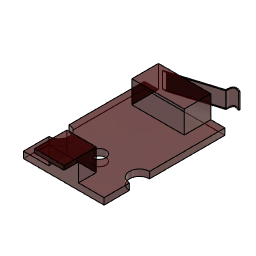
Rover base v7 (Autodesk Fusion 360 archive; units mm, degrees)
design "Crash sensor"
Autodesk Fusion 360 part; units mm, degrees
sketch "Sketch1" plane through (0, 0, 0) normal (0, 0, 1) x (1, 0, 0)
  line L0 (10, -15) -> (-10, -15)
  line L1 (-10, -15) -> (-10, 15)
  line L2 (-10, 15) -> (10, 15)
  line L3 (10, 15) -> (10, -15)
  line L4 (10, -15) -> (-10, 15) construction
  line L5 (-10, -15) -> (10, 15) construction
  dimension "d1" = 20
  dimension "d2" = 30
  constraint horizontal L0
  constraint perpendicular L0 L1
  constraint parallel L0 L2
  constraint parallel L1 L3
  constraint coincident L4 origin
  constraint coincident L5 origin
  measures "d1" distance of L1.end L2.end
  measures "d2" distance of L0.start L2.end
extrude "Extrude1" add sketch "Sketch1" along normal blind 1.6
sketch "Sketch2" plane through (0, 0, 1.6) normal (0, 0, 1) x (-1, 0, 0)
  line L0 (-10, -15) -> (10, -15)
  line L1 (10, -15) -> (10, 15)
  line L2 (10, 15) -> (-10, 15)
  line L3 (-10, 15) -> (-10, -15)
  line L4 (6.5, -15) -> (-6.5, -15)
  line L5 (-6.5, -15) -> (-6.5, -8.4)
  line L6 (-6.5, -8.4) -> (6.5, -8.4)
  line L7 (6.5, -8.4) -> (6.5, -15)
  point P0 (0, -8.4)
  dimension "d5" = 13
  dimension "d6" = 6.6
  constraint horizontal L4
  constraint vertical L5
  constraint horizontal L6
  constraint vertical L7
  constraint midpoint L6 P0
  constraint vertical origin P0
  constraint collinear L0 L4
  measures "d5" distance of L4.start L4.end
  measures "d6" distance of L4.end L5.end
extrude "Extrude2" add sketch "Sketch2" along normal blind 5.6 contours L0 L4 L5 L6 L7
sketch "Sketch3" plane through (0, 0, 7.2) normal (0, 0, 1) x (-1, 0, 0)
  line L0 (6.5, -8.4) -> (-6.5, -8.4)
  line L1 (-6.5, -8.4) -> (-6.5, -15)
  line L2 (-6.5, -15) -> (6.5, -15)
  line L3 (6.5, -15) -> (6.5, -8.4)
  line L4 (5.5056, -15) -> (-6.5, -18.7)
  spline S0 degree 5 poles (-6.5, -18.7) (-6.4971, -18.7969) (-6.4951, -18.9849) (-6.504, -19.2489) (-6.5399, -19.5646) (-6.6275, -19.8945) (-6.7616, -20.154) (-6.9462, -20.3373) (-7.1832, -20.441) (-7.4708, -20.4684) (-7.8051, -20.4252) (-8.1068, -20.3387) (-8.3512, -20.2464) (-8.522, -20.173) (-8.6094, -20.1333) knots 0 0 0 0 0 0 0.1 0.2 0.3 0.4 0.5 0.6 0.7 0.8 0.9 1 1 1 1 1 1
  line L5 (5.4173, -14.7133) -> (-6.8068, -18.4806)
  spline S1 degree 3 poles (-6.8068, -18.4806) (-6.8045, -18.5568) (-6.8022, -18.6329) (-6.7999, -18.7091) (-6.7803, -19.3532) (-6.8883, -19.803) (-7.0372, -19.9851) (-7.1506, -20.1238) (-7.2845, -20.1741) (-7.572, -20.1446) (-7.8085, -20.1203) (-8.1221, -20.0252) (-8.4853, -19.8601) knots -0.047137 -0.047137 -0.047137 -0.047137 0 0 0 0.418701 0.418701 0.418701 0.737623 0.737623 0.737623 1 1 1 1
  line L6 (-8.4853, -19.8601) -> (-8.6094, -20.1333)
  line L7 (5.4173, -14.7133) -> (5.5056, -15)
  point P0 (-6.9617, -20.3191)
  dimension "d9" = 3.7
  dimension "d10" = 0.3
  constraint coincident L2 L4.start
  constraint perpendicular L4 L7
  measures "d9" distance of L1.end L4.end
extrude "Extrude3" add sketch "Sketch3" against normal blind 4 from surface at -1 contours L2 L4 S0 L5 S1 L6
sketch "Sketch4" plane through (0, 0, 1.6) normal (0, 0, 1) x (-1, 0, 0)
  line L0 (-6.5, -15) -> (-6.5, -8.4)
  line L1 (-6.5, -8.4) -> (6.5, -8.4)
  line L2 (6.5, -8.4) -> (6.5, -15)
  line L3 (6.5, -15) -> (10, -15)
  line L4 (10, -15) -> (10, 15)
  line L5 (10, 15) -> (-10, 15)
  line L6 (-10, 15) -> (-10, -15)
  line L7 (-10, -15) -> (-6.5, -15)
  circle A0 centre (-10, 6.2) radius 2.5
  circle A1 centre (10, 6.2) radius 2.5
  circle A2 centre (0, 6.2) radius 1.65
  dimension "d14" = 5
  dimension "d15" = 5
  dimension "d16" = 8.8
  dimension "d17" = 8.8
  dimension "d18" = 3.3
  dimension "d19" = 8.8
  constraint coincident L6 A0.centre
  constraint coincident L4 A1.centre
  constraint vertical origin A2.centre
  measures "d14" diameter of A0
  measures "d15" diameter of A1
  measures "d16" distance of L5.end A0.centre
  measures "d17" distance of L4.end A1.centre
  measures "d18" diameter of A2
  measures "d19" distance of L5 A2.centre
extrude "Extrude4" cut sketch "Sketch4" against normal blind 6 contours L6 A0 | L4 A1 | A2 picked at (-9.2516, 6.7372) picked at (8.4513, 6.9963)
sketch "Sketch5" plane through (0, 0, 1.6) normal (0, 0, 1) x (-1, 0, 0)
  arc A0 (-10, 3.7) -> (-10, 8.7) centre (-10, 6.2) ccw
  line L0 (-10, 3.7) -> (-10, -15)
  line L1 (-10, -15) -> (-6.5, -15)
  line L2 (-6.5, -15) -> (-6.5, -8.4)
  line L3 (-6.5, -8.4) -> (6.5, -8.4)
  line L4 (6.5, -8.4) -> (6.5, -15)
  line L5 (6.5, -15) -> (10, -15)
  line L6 (10, -15) -> (10, 3.7)
  arc A1 (10, 8.7) -> (10, 3.7) centre (10, 6.2) ccw
  line L7 (10, 8.7) -> (10, 15)
  line L8 (10, 15) -> (-10, 15)
  line L9 (-10, 15) -> (-10, 8.7)
  circle A2 centre (0, 6.2) radius 1.65
  line L10 (3.65, 15) -> (-3.65, 15)
  line L11 (-3.65, 15) -> (-3.65, 10.58)
  line L12 (-3.65, 10.58) -> (3.65, 10.58)
  line L13 (3.65, 10.58) -> (3.65, 15)
  point P0 (0, 10.58)
  dimension "d22" = 4.42
  dimension "d23" = 7.3
  constraint horizontal L10
  constraint vertical L11
  constraint horizontal L12
  constraint vertical L13
  constraint coincident L8 L10.start
  constraint midpoint L12 P0
  constraint vertical origin P0
  measures "d2" distance of L0.end
  measures "d22" distance of L10.end L11.end
  measures "d23" distance of L10.start L10.end
extrude "Extrude5" add sketch "Sketch5" along normal blind 5.5 contours L8 L10 L11 L12 L13
sketch "Sketch6" plane through (0, 0, 7.1) normal (0, 0, 1) x (-1, 0, 0)
  line L0 (3.65, 10.58) -> (3.65, 15)
  line L1 (3.65, 15) -> (-3.65, 15)
  line L2 (-3.65, 15) -> (-3.65, 10.58)
  line L3 (-3.65, 10.58) -> (3.65, 10.58)
  line L4 (3.65, 10.58) -> (-3.65, 10.58)
  line L5 (-3.65, 10.58) -> (-3.65, 18.58)
  line L6 (-3.65, 18.58) -> (3.65, 18.58)
  line L7 (3.65, 18.58) -> (3.65, 10.58)
  dimension "d26" = 8
  constraint horizontal L4
  constraint vertical L5
  constraint horizontal L6
  constraint vertical L7
  constraint coincident L0.start L3.end
  constraint collinear L2 L5
  measures "d26" distance of L4 L6
extrude "Extrude6" add sketch "Sketch6" against normal blind 1 contours L1 L5 L6 L7

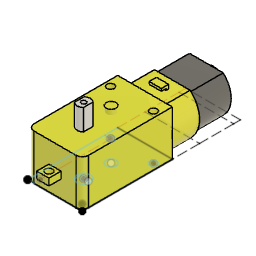
design "Yellow Gearbox motor v3"
Autodesk Fusion 360 part; units mm, degrees
sketch "Sketch1" plane through (0, 0, 0) normal (0, 0, 1) x (1, 0, 0) in component "Yellow TT Motor"
  line L0 (2.555, 0) -> (19.885, 0)
  line L1 (22.44, 2.555) -> (22.44, 37)
  line L2 (22.44, 37) -> (0, 37)
  line L3 (0, 37) -> (0, 2.555)
  arc A0 (19.885, 0) -> (22.44, 2.555) centre (19.885, 2.555) ccw
  arc A1 (0, 2.555) -> (2.555, 0) centre (2.555, 2.555) ccw
  line L4 (2.555, 2.555) -> (2.555, 11.805) construction
  circle A2 centre (11.22, 11.805) radius 0.975
  circle A3 centre (11.22, 11.805) radius 2.7
  line L5 (11.22, 11.805) -> (13.07, 11.805) construction
  line L6 (13.0698, 9.8382) -> (13.0698, 13.7718)
  line L7 (9.3702, 9.8382) -> (9.3702, 13.7718)
  line L8 (2.555, 11.805) -> (2.555, 23.055) construction
  line L9 (2.555, 23.055) -> (2.555, 31.655) construction
  line L10 (0, 31.655) -> (2.42, 31.655) construction
  line L11 (22.44, 31.655) -> (20.02, 31.655) construction
  circle A4 centre (2.42, 31.655) radius 1.5
  circle A5 centre (20.02, 31.655) radius 1.5
  circle A6 centre (11.22, 23.055) radius 2
  line L12 (0, 37) -> (0, 48.2) construction
  line L13 (0, 48.2) -> (22.44, 48.2) construction
  line L14 (22.44, 48.2) -> (22.44, 37) construction
  line L15 (0, 48.2) -> (0, 62.2) construction
  line L16 (0, 62.2) -> (22.44, 62.2) construction
  line L17 (22.44, 62.2) -> (22.44, 48.2) construction
  line L18 (22.44, 62.2) -> (22.44, 65) construction
  line L19 (22.44, 65) -> (0, 65) construction
  line L20 (0, 65) -> (0, 62.2) construction
  point P0 (22.44, 0)
  dimension "d1" = 22.44
  dimension "d2" = 37
  dimension "d3" = 2.555
  dimension "d5" = 9.25
  dimension "d6" = 1.95
  dimension "d7" = 5.4
  dimension "d8" = 1.85
  dimension "d10" = 11.25
  dimension "d11" = 8.6
  dimension "d13" = 2.42
  dimension "d14" = 3
  dimension "d15" = 3
  dimension "d16" = 4
  dimension "d28" = 11.2
  dimension "d29" = 14
  dimension "d45" = 2.8
  constraint horizontal L0
  constraint perpendicular L0 L1
  constraint perpendicular L1 L2
  constraint perpendicular L0 L3
  constraint coincident P0 L1
  constraint coincident P0 L0
  constraint tangent L1 A0
  constraint tangent L0 A0
  constraint coincident origin L0
  constraint tangent L3 A1
  constraint tangent L0 A1
  constraint equal A0 A1
  constraint coincident A1.centre L4.start
  constraint parallel L3 L4
  constraint concentric A2 A3
  constraint coincident A2.centre A3.centre
  constraint coincident A3 L6.start
  constraint coincident A3 L6.end
  constraint coincident A3 L7.start
  constraint coincident A3 L7.end
  constraint parallel L6 L7
  constraint parallel L3 L8
  constraint parallel L8 L9
  constraint coincident L3 L10.start
  constraint coincident L1 L11.start
  constraint perpendicular L9 L10
  constraint perpendicular L1 L11
  constraint coincident L10.end A4.centre
  constraint coincident L11.end A5.centre
  constraint perpendicular L2 L12
  constraint perpendicular L1 L13
  constraint perpendicular L2 L14
  constraint perpendicular L13 L15
  constraint perpendicular L14 L16
  constraint perpendicular L13 L17
  constraint perpendicular L16 L18
  constraint perpendicular L18 L19
  constraint perpendicular L16 L20
  measures "d1" distance of origin P0
  measures "d2" distance of P0 L1.end
  measures "d3" radius of A0
  measures "d5" distance of A1.centre L4.end
  measures "d6" diameter of A2
  measures "d7" diameter of A3
  measures "d8" distance of A2.centre L5.end
  measures "d10" distance of L4.end L8.end
  measures "d11" distance of L8.end L9.end
  measures "d13" distance of L11.start L11.end
  measures "d14" diameter of A4
  measures "d15" diameter of A5
  measures "d16" diameter of A6
  measures "d28" distance of L2.end L12.end
  measures "d29" distance of L12.end L15.end
  measures "d45" distance of L16.end L18.end
extrude "Extrude2" add sketch "Sketch1" along normal blind 20.52 contours A6 makes body 1 in component "Yellow TT Motor"
extrude "Extrude1" add sketch "Sketch1" along normal blind 18.6 separate body contours L0 L1 L2 L3 A0 A1 | A2 | A3 L6 | A3 L6 L7 | A3 L7 | A6 makes body 2 in component "Yellow TT Motor"
extrude "Extrude3" add sketch "Sketch1" against normal blind 9.3 contours A3 L6 L7 bodies 2 in component "Yellow TT Motor"
extrude "Extrude4" add 1 faces at (9.6618, 11.805, -9.3) along direction (0, 0, 1) blind 36.6 on bodies 2 bodies 2 in component "Yellow TT Motor"
extrude "Extrude5" add sketch "Sketch1" against normal blind 1.92 contours A3 L6 | A3 L7 bodies 2 in component "Yellow TT Motor"
sketch "Sketch5" plane through (0, 37, 0) normal (0, 1, 0) x (-1, 0, 0)
  line L0 (-22.44, 0) -> (0, 0)
  line L1 (0, 0) -> (0, 18.6)
  line L2 (0, 18.6) -> (-22.44, 18.6)
  line L3 (-22.44, 18.6) -> (-22.44, 0)
  line L4 (0, 0) -> (0, 17) construction
  line L5 (0, 17) -> (-22.44, 17) construction
  line L6 (-11.22, 17) -> (-11.22, 0) construction
  circle A0 centre (-11.22, 8.5) radius 11.22 construction
  arc A1 (-3.8962, 0) -> (-3.8962, 17) centre (-11.22, 8.5) ccw
  arc A2 (-18.5438, 17) -> (-18.5438, 0) centre (-11.22, 8.5) ccw
  line L7 (-18.5438, 0) -> (-3.8962, 0)
  line L8 (-3.8962, 17) -> (-18.5438, 17)
  constraint coincident L0.end L1.start
  constraint coincident L1 L4.end
  constraint perpendicular L0 L4
  constraint coincident L3 L5.end
  constraint perpendicular L3 L5
  constraint midpoint L5 L6.start
  constraint midpoint L0 L6.end
  constraint tangent L3 A0
  constraint coincident A0 A1.end
  constraint coincident L5 A1.end
  constraint coincident A0 A1.start
  constraint coincident L0 A1.start
  constraint coincident A0.centre A1.centre
  constraint coincident A0 A2.end
  constraint coincident L0 A2.end
  constraint parallel L5 L8
extrude "Extrude6" add sketch "Sketch5" along normal blind 11.2 contours L0 A1 A2 L7 L8 bodies 2 in component "Yellow TT Motor"
sketch "Sketch6" plane through (0, 48.2, 0) normal (0, 1, 0) x (-1, 0, 0)
  line L0 (-3.8962, 17) -> (-18.5438, 17)
  arc A0 (-18.5438, 17) -> (-18.5438, 0) centre (-11.22, 8.5) ccw
  line L1 (-18.5438, 0) -> (-3.8962, 0)
  arc A1 (-3.8962, 0) -> (-3.8962, 17) centre (-11.22, 8.5) ccw
  line L2 (-18.1625, 1) -> (-4.2775, 1)
  arc A2 (-4.2775, 1) -> (-4.2775, 16) centre (-11.22, 8.5) ccw
  line L3 (-4.2775, 16) -> (-18.1625, 16)
  arc A3 (-18.1625, 16) -> (-18.1625, 1) centre (-11.22, 8.5) ccw
  dimension "d33" = -1
extrude "Extrude7" add sketch "Sketch6" along normal blind 14 contours L2 A2 L3 A3 bodies 2 in component "Yellow TT Motor"
sketch "Sketch7" plane through (0, 0, 0) normal (0, -1, 0) x (1, 0, 0)
  line L0 (2.555, 0) -> (19.885, 0)
  line L1 (19.885, 0) -> (19.885, 18.6)
  line L2 (19.885, 18.6) -> (2.555, 18.6)
  line L3 (2.555, 18.6) -> (2.555, 0)
  line L4 (11.22, 0) -> (11.22, 17) construction
  line L5 (11.22, 17) -> (19.885, 17) construction
  line L6 (11.22, 17) -> (2.555, 17) construction
  line L7 (11.22, 1.9503) -> (13.72, 1.9503) construction
  line L8 (11.22, 1.9503) -> (8.72, 1.9503) construction
  line L9 (13.72, 1.9503) -> (13.72, 17) construction
  line L10 (8.72, 1.9503) -> (8.72, 17) construction
  line L11 (11.22, 8.5) -> (11.22, 9.9) construction
  line L12 (8.72, 9.9) -> (13.72, 9.9)
  line L13 (13.72, 9.9) -> (13.72, 7.1)
  line L14 (13.72, 7.1) -> (8.72, 7.1)
  line L15 (8.72, 7.1) -> (8.72, 9.9)
  dimension "d36" = 17
  dimension "d37" = 2.5
  dimension "d38" = 2.5
  dimension "d39" = 1.4
  constraint midpoint L0 L4.start
  constraint perpendicular L0 L4
  constraint coincident L1 L5.end
  constraint perpendicular L1 L5
  constraint coincident L3 L6.end
  constraint perpendicular L3 L6
  constraint coincident L4 L7.start
  constraint perpendicular L4 L7
  constraint perpendicular L4 L8
  constraint perpendicular L7 L9
  constraint coincident L6 L10.end
  constraint perpendicular L6 L10
  constraint midpoint L4 L11.start
  constraint perpendicular L6 L11
  constraint coincident L10 L12.start
  constraint coincident L9 L12.end
  constraint perpendicular L9 L12
  constraint coincident L9 L13.end
  constraint coincident L10 L14.end
  constraint perpendicular L10 L14
  constraint perpendicular L12 L15
  measures "d36" distance of L4.start L4.end
  measures "d37" distance of L7.start L7.end
  measures "d38" distance of L7.start L8.end
  measures "d39" distance of L11.start L11.end
extrude "Extrude8" add sketch "Sketch7" along normal blind 5 contours L12 L13 L14 L15 bodies 2 in component "Yellow TT Motor"
sketch "Sketch8" plane through (0, 0, 9.9) normal (0, 0, 1) x (-1, 0, 0)
  line L0 (-13.72, 0) -> (-8.72, 0)
  line L1 (-8.72, 0) -> (-8.72, 5)
  line L2 (-8.72, 5) -> (-13.72, 5)
  line L3 (-13.72, 5) -> (-13.72, 0)
  line L4 (-8.72, 5) -> (-13.72, 0) construction
  circle A0 centre (-11.22, 2.5) radius 1.5
  dimension "d42" = 3
  constraint coincident L1.end L2.start
  constraint coincident L0.start L3.end
  constraint midpoint L4 A0.centre
  measures "d42" diameter of A0
extrude "Extrude9" cut sketch "Sketch8" against normal blind 3 contours A0 bodies 2 in component "Yellow TT Motor"
sketch "Sketch9" plane through (0, 62.2, 0) normal (0, 1, 0) x (-1, 0, 0)
  arc A0 (-18.1625, 16) -> (-18.1625, 1) centre (-11.22, 8.5) ccw
  line L0 (-18.1625, 1) -> (-4.2775, 1)
  arc A1 (-4.2775, 1) -> (-4.2775, 16) centre (-11.22, 8.5) ccw
  line L1 (-4.2775, 16) -> (-18.1625, 16)
  line L2 (-1, 8.5) -> (-21.44, 8.5) construction
  line L3 (-11.22, 16) -> (-11.22, 1) construction
  circle A2 centre (-11.22, 8.5) radius 5 construction
  line L4 (-11.22, 13.5) -> (-11.22, 4.5) construction
  line L5 (-14.2758, 4.5424) -> (-8.1642, 4.5424)
  arc A3 (-8.1642, 4.5424) -> (-14.2758, 4.5424) centre (-11.22, 8.5) ccw
  dimension "d46" = 10
  constraint midpoint A1 L2.start
  constraint midpoint A0 L2.end
  constraint midpoint L1 L3.start
  constraint midpoint L0 L3.end
  constraint concentric A0 A2
  constraint coincident L3 L4.start
  constraint coincident A2 L4.start
  constraint parallel L3 L4
  constraint coincident A2 L5.start
  constraint coincident A2 L5.end
  constraint perpendicular L4 L5
  constraint coincident A0.centre A1.centre
  measures "d46" diameter of A2
extrude "Extrude10" add sketch "Sketch9" along normal blind 2.8 contours L5 A3 bodies 2 in component "Yellow TT Motor"
sketch "Sketch10" plane through (0, 0, 17) normal (0, 0, 1) x (-1, 0, 0)
  line L0 (-3.8962, -37) -> (-18.5438, -37)
  line L1 (-18.5438, -37) -> (-18.5438, -48.2)
  line L2 (-18.5438, -48.2) -> (-3.8962, -48.2)
  line L3 (-3.8962, -48.2) -> (-3.8962, -37)
  line L4 (-11.22, -48.2) -> (-11.22, -44.2) construction
  line L5 (-11.22, -44.2) -> (-8.72, -44.2)
  line L6 (-8.72, -44.2) -> (-13.72, -44.2)
  line L7 (-8.72, -44.2) -> (-8.72, -43.2)
  line L8 (-8.72, -43.2) -> (-13.72, -43.2)
  line L9 (-13.72, -43.2) -> (-13.72, -44.2)
  dimension "d50" = 4
  dimension "d52" = 5
  dimension "d53" = 1
  constraint midpoint L2 L4.start
  constraint perpendicular L2 L4
  constraint perpendicular L4 L5
  constraint perpendicular L4 L6
  constraint perpendicular L5 L7
  constraint perpendicular L7 L8
  constraint perpendicular L6 L9
  measures "d50" distance of L4.start L4.end
  measures "d52" distance of L5.end L6.end
  measures "d53" distance of L5.end L7.end
extrude "Extrude11" add sketch "Sketch10" along normal blind 1.7 contours L5 L6 L7 L8 L9 bodies 2 in component "Yellow TT Motor"
sketch "Sketch11" plane through (0, 43.2, 0) normal (0, -1, 0) x (1, 0, 0)
  line L0 (8.72, 17) -> (13.72, 17)
  line L1 (13.72, 17) -> (13.72, 18.7)
  line L2 (13.72, 18.7) -> (8.72, 18.7)
  line L3 (8.72, 18.7) -> (8.72, 17)
  line L4 (11.22, 18.7) -> (11.22, 17.7) construction
  line L5 (13.72, 17.7) -> (8.72, 17.7)
  dimension "d56" = 1
  constraint midpoint L2 L4.start
  constraint perpendicular L2 L4
  constraint coincident L1 L5.start
  constraint coincident L3 L5.end
  constraint perpendicular L3 L5
  measures "d56" distance of L4.start L4.end
extrude "Extrude12" add sketch "Sketch11" along normal blind 2 contours L1 L2 L3 L5 bodies 2 in component "Yellow TT Motor"
sketch "Sketch12" plane through (0, 0, 0) normal (0, 0, -1) x (1, 0, 0)
  circle A0 centre (11.22, -11.805) radius 2.7
  arc A1 (2.555, 0) -> (0, -2.555) centre (2.555, -2.555) ccw
  line L0 (0, -2.555) -> (0, -37)
  line L1 (0, -37) -> (3.8962, -37)
  line L2 (3.8962, -37) -> (3.8962, -48.2)
  line L3 (3.8962, -48.2) -> (18.5438, -48.2)
  line L4 (18.5438, -48.2) -> (18.5438, -37)
  line L5 (18.5438, -37) -> (22.44, -37)
  line L6 (22.44, -37) -> (22.44, -2.555)
  arc A2 (22.44, -2.555) -> (19.885, 0) centre (19.885, -2.555) ccw
  line L7 (19.885, 0) -> (2.555, 0)
  circle A3 centre (20.02, -31.655) radius 1.5
  circle A4 centre (2.42, -31.655) radius 1.5
  line L8 (8.72, -44.2) -> (13.72, -44.2)
  line L9 (13.72, -44.2) -> (13.72, -43.2)
  line L10 (13.72, -43.2) -> (8.72, -43.2)
  line L11 (8.72, -43.2) -> (8.72, -44.2)
  line L12 (3.8962, -37) -> (18.5438, -37)
  line L13 (18.5438, -37) -> (18.5438, -48.2)
  line L14 (18.5438, -48.2) -> (3.8962, -48.2)
  line L15 (3.8962, -48.2) -> (3.8962, -37)
  line L16 (8.72, -44.2) -> (13.72, -44.2)
  line L17 (13.72, -44.2) -> (13.72, -43.2)
  line L18 (13.72, -43.2) -> (8.72, -43.2)
  line L19 (8.72, -43.2) -> (8.72, -44.2)
extrude "Extrude13" add sketch "Sketch12" along normal blind 1.7 contours L8 L9 L10 L11 L16 L17 L18 L19 bodies 2 in component "Yellow TT Motor"
sketch "Sketch13" plane through (0, 43.2, 0) normal (0, -1, 0) x (1, 0, 0)
  line L0 (13.72, 0) -> (8.72, 0)
  line L1 (8.72, 0) -> (8.72, -1.7)
  line L2 (8.72, -1.7) -> (13.72, -1.7)
  line L3 (13.72, -1.7) -> (13.72, 0)
  line L4 (11.22, -1.7) -> (11.22, -0.7) construction
  line L5 (8.72, -0.7) -> (13.72, -0.7)
  line L6 (8.72, -0.7) -> (8.72, -1.7)
  line L7 (8.72, -1.7) -> (13.72, -1.7)
  line L8 (13.72, -0.7) -> (13.72, -1.7)
  dimension "d61" = 1
  constraint midpoint L2 L4.start
  constraint perpendicular L2 L4
  constraint coincident L1 L5.start
  constraint coincident L3 L5.end
  constraint perpendicular L3 L5
  constraint coincident L1.end L2.start
  constraint perpendicular L2 L6
  constraint coincident L2.end L3.start
  measures "d61" distance of L4.start L4.end
extrude "Extrude14" add sketch "Sketch13" along normal blind 2 contours L1 L2 L3 L5 L6 L7 L8 bodies 2 in component "Yellow TT Motor"
component "Yellow TT Motor" placed x (1, 0, 0) y (0, 1, 0) z (0, 0, 1) at (0, 0, 0)
